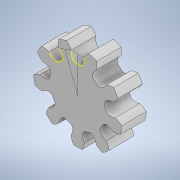
# Autodesk Inventor part: SmallGear9T
Saved by Autodesk Inventor 2022 (Build 260153070, 153G)
## iProperties
Created: 2021-11-03
Part Number: SmallGear9T
Material: Generic
Document SubType Name: Modeling
Designer: a laptop
Density: 1 g/cm^3
Appearance: Default
Author: a laptop
Autodesk Inventor part; units mm, degrees
ref_plane "YZ Plane" through (0, 0, 0) normal (1, 0, 0) x (0, 1, 0)
ref_plane "XZ Plane" through (0, 0, 0) normal (0, 1, 0) x (-1, 0, 0)
ref_plane "XY Plane" through (0, 0, 0) normal (0, 0, 1) x (1, 0, 0)
sketch "Sketch1" plane through (0, 0, 0) normal (0, 0, 1) x (1, 0, 0)
  spline S0 degree 3 poles (-1.3464, 5.2146) (-1.2887, 5.1626) (-1.1733, 5.0587) (-1.0189, 4.8841) (-0.8785, 4.6973) (-0.8096, 4.558) (-0.7752, 4.4884) knots 0 0 0 0 0.250071 0.500149 0.750165 1 1 1 1
  spline S1 degree 3 poles (-0.7752, 4.4884) (-0.7857, 4.4211) (-0.8066, 4.2867) (-0.8068, 4.0817) (-0.7737, 3.8799) (-0.7064, 3.686) (-0.5864, 3.5181) (-0.4401, 3.4219) (-0.3061, 3.3934) (-0.1697, 3.3977) (0, 3.4077) (0.1697, 3.3977) (0.3061, 3.3934) (0.4401, 3.4219) (0.5864, 3.5181) (0.7064, 3.686) (0.7737, 3.8799) (0.8068, 4.0817) (0.8066, 4.2867) (0.7857, 4.4211) (0.7752, 4.4884) knots 0 0 0 0 0.062606 0.125231 0.187814 0.250234 0.312597 0.374754 0.406093 0.437398 0.5 0.562602 0.593907 0.625246 0.687403 0.749766 0.812186 0.874769 0.937394 1 1 1 1
  spline S2 degree 3 poles (0.7752, 4.4884) (0.8096, 4.558) (0.8785, 4.6973) (1.0189, 4.8841) (1.1733, 5.0587) (1.2887, 5.1626) (1.3464, 5.2146) knots 0 0 0 0 0.249835 0.499851 0.749929 1 1 1 1
  circle A0 centre (0, 0) radius 3.4037 construction
  circle A1 centre (0, 0) radius 4.4316 construction
  circle A2 centre (0, 0) radius 4.5 construction
  circle A3 centre (0, 0) radius 5.3856
  point P0 (-1.1764, 5.0556)
  point P1 (-1.0212, 4.882)
  point P2 (-0.8847, 4.6936)
  point P3 (-0.8014, 4.2861)
  point P4 (-0.8012, 4.0821)
  point P5 (-0.7679, 3.881)
  point P6 (-0.6976, 3.6902)
  point P7 (-0.577, 3.5267)
  point P8 (-0.4056, 3.4189)
  point P9 (-0.3058, 3.3975)
  point P10 (-0.2038, 3.3969)
  point P11 (0, 3.4037)
  point P12 (0.2038, 3.3969)
  point P13 (0.3058, 3.3975)
  point P14 (0.4056, 3.4189)
  point P15 (0.577, 3.5267)
  point P16 (0.6976, 3.6902)
  point P17 (0.7679, 3.881)
  point P18 (0.8012, 4.0821)
  point P19 (0.8014, 4.2861)
  point P20 (0.8847, 4.6936)
  point P21 (1.0212, 4.882)
  point P22 (1.1764, 5.0556)
  constraints: 4 centre point, 2 point on circle, 61 other
extrude "Extrusion1" add sketch "Sketch1" against normal blind 3
extrude "Extrusion2" cut sketch "Sketch1" against normal blind 10 contours A3 S2 S1 S0 picked at (0.151, 4.7811)
pattern_circular "Circular Pattern1" count 9 over 360 about axis through (0, 0, 0) along (0, 0, -1) of "Extrusion2"
sketch "Sketch2" plane through (0, 0, 0) normal (0, 0, 1) x (1, 0, 0)
  line L0 (-2.2912, 3.9366) -> (-0.7752, 4.4884) construction
  line L1 (0.7752, 4.4884) -> (-0.7752, 4.4884) construction
  line L2 (-1.5332, 4.2125) -> (0, 0) construction
  line L3 (0, 0) -> (0, 4.4884) construction
  constraints: 8 end point, 2 midpoint, 1 horizontal, 1 horizontal alignment, 1 other
equation "\"d0\" = FaceWidth"
equation "\"Module\" = 1"
equation "\"PressureAngle\" = 10deg"
equation "\"UnitProfileClearance\" = 0.25"
equation "\"UnitRoundRadius\" = 0.3025"
equation "\"HeadDiameter\" = 10.77128"
equation "\"RootDiameter\" = 6.80735"
equation "\"BaseDiameter\" = 8.86327"
equation "\"PitchDiameter\" = 9"
equation "\"FaceWidth\" = 3"
equation "\"HelixAngle\" = 0"
equation "\"UnitCorrection\" = 0.153676"
equation "\"UnitAddendumModification\" = 0.268038"
equation "\"CircularPitch\" = 3.141593"
equation "\"UnitBacklashShift\" = 0"
equation "\"TotalToolShift\" = 0.15368"
equation "\"IsInternal\" = 0"
body "Solid1"
